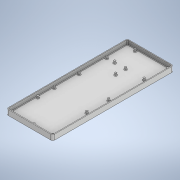
# Autodesk Inventor part: Base
Saved by Autodesk Inventor 2022 (Build 260153000, 153)
## iProperties
Created: 2021-09-21
Part Number: Base
Material: 一般
Document SubType Name: Modeling
Designer: shiok
Density: 1 g/cm^3
Appearance: 既定
Author: shiok
Autodesk Inventor part; units mm, degrees
ref_plane "YZ Plane" through (0, 0, 0) normal (1, 0, 0) x (0, 1, 0)
ref_plane "XZ Plane" through (0, 0, 0) normal (0, 1, 0) x (-1, 0, 0)
ref_plane "XY Plane" through (0, 0, 0) normal (0, 0, 1) x (1, 0, 0)
sketch "スケッチ1" plane through (0, 0, 0) normal (0, 1, 0) x (-1, 0, 0)
  line L0 (65.58, 183.1975) -> (-65.58, 183.1975)
  line L1 (-68.58, 180.1975) -> (-68.58, -180.1975)
  line L2 (-65.58, -183.1975) -> (65.58, -183.1975)
  line L3 (68.58, -180.1975) -> (68.58, 180.1975)
  arc A0 (68.58, 180.1975) -> (65.58, 183.1975) centre (65.58, 180.1975) ccw
  arc A1 (65.58, -183.1975) -> (68.58, -180.1975) centre (65.58, -180.1975) ccw
  arc A2 (-68.58, -180.1975) -> (-65.58, -183.1975) centre (-65.58, -180.1975) ccw
  arc A3 (-65.58, 183.1975) -> (-68.58, 180.1975) centre (-65.58, 180.1975) ccw
  line L4 (71.12, 180.1975) -> (71.12, -180.1975)
  arc A4 (65.58, -185.7375) -> (71.12, -180.1975) centre (65.58, -180.1975) ccw
  line L5 (65.58, -185.7375) -> (-65.58, -185.7375)
  arc A5 (-71.12, -180.1975) -> (-65.58, -185.7375) centre (-65.58, -180.1975) ccw
  line L6 (-71.12, -180.1975) -> (-71.12, 180.1975)
  arc A6 (-65.58, 185.7375) -> (-71.12, 180.1975) centre (-65.58, 180.1975) ccw
  line L7 (-65.58, 185.7375) -> (65.58, 185.7375)
  arc A7 (71.12, 180.1975) -> (65.58, 185.7375) centre (65.58, 180.1975) ccw
  line L8 (-65.58, 180.1975) -> (65.58, -180.1975) construction
  line L9 (-65.58, -180.1975) -> (65.58, 180.1975) construction
  circle A8 centre (62.23, 176.8475) radius 3
  circle A9 centre (63.5, 96.8375) radius 3
  circle A10 centre (63.5, 46.0375) radius 3
  circle A11 centre (62.23, -28.8925) radius 3
  circle A12 centre (62.23, -113.9825) radius 3
  circle A13 centre (38.1, -113.9825) radius 3
  circle A14 centre (38.1, -176.8475) radius 3
  circle A15 centre (-62.23, -176.8475) radius 3
  circle A16 centre (4.445, -113.9825) radius 3
  circle A17 centre (4.445, -83.5025) radius 3
  circle A18 centre (-52.705, -113.9825) radius 3
  circle A19 centre (-52.705, -4.7625) radius 3
  circle A20 centre (-52.705, 62.4375) radius 3
  circle A21 centre (-62.23, 176.8475) radius 3
  circle A22 centre (-5.08, 176.8475) radius 3
  point P0 (0, 0)
  point P1 (0, 0)
  point P2 (0, 0)
  point P3 (52.07, 166.6875)
  dimension "d2" = 3
  dimension "d3" = 2.54
  dimension "d5" = 366.395
  dimension "d6" = 137.16
  dimension "d7" = 16.51
  dimension "d8" = 16.51
  dimension "d9" = 10.16
  dimension "d10" = 10.16
  dimension "d11" = 1.27
  dimension "d12" = 1.27
  dimension "d13" = 80.01
  dimension "d14" = 50.8
  dimension "d15" = 74.93
  dimension "d16" = 85.09
  dimension "d17" = 6
  dimension "d18" = 6
  dimension "d19" = 6
  dimension "d20" = 6
  dimension "d21" = 6
  dimension "d22" = 24.13
  dimension "d23" = 62.865
  dimension "d24" = 100.33
  dimension "d25" = 62.865
  dimension "d26" = 9.525
  dimension "d27" = 6
  dimension "d28" = 6
  dimension "d29" = 57.15
  dimension "d30" = 67.2
  dimension "d31" = 6
  dimension "d32" = 6
  dimension "d33" = 109.22
  dimension "d34" = 6
  dimension "d35" = 6
  dimension "d36" = 6
  dimension "d37" = 6
  dimension "d38" = 6
  dimension "d39" = 6
  dimension "d40" = 30.48
  dimension "d41" = 33.655
  constraints: 23 centre point, 20 end point, 16 point on circle, 8 tangent, 7 vertical alignment, 5 horizontal alignment, 4 parallel, 3 equal radius, 3 midpoint, 2 perpendicular, 1 coincident, 1 horizontal, 7 other
  measures "d2" radius of A0
  measures "d3" distance between parallel lines of L3 L4
  measures "d5" distance between parallel lines of L2 L0
  measures "d6" distance between parallel lines of L1 L3
  measures "d7" distance from line of point (52.07, 166.688) L3
  measures "d8" distance from line of L0 point (52.07, 166.688)
  measures "d9" horizontal distance of A8.centre point (52.07, 166.688)
  measures "d10" horizontal distance of point (52.07, 166.688) A8.centre
  measures "d11" horizontal distance of A9.centre A8.centre
  measures "d12" horizontal distance of A11.centre A10.centre
  measures "d13" vertical distance of A9.centre A8.centre
  measures "d14" distance of A9.centre A10.centre
  measures "d15" vertical distance of A10.centre A11.centre
  measures "d16" distance of A12.centre A11.centre
  measures "d17" diameter of A8
  measures "d18" diameter of A9
  measures "d19" diameter of A10
  measures "d20" diameter of A11
  measures "d21" diameter of A12
  measures "d22" distance of A13.centre A12.centre
  measures "d23" distance of A14.centre A13.centre
  measures "d24" distance of A15.centre A14.centre
  measures "d25" vertical distance of A18.centre A15.centre
  measures "d26" horizontal distance of A18.centre A15.centre
  measures "d27" diameter of A21
  measures "d28" diameter of A22
  measures "d29" distance of A21.centre A22.centre
  measures "d30" distance of A19.centre A20.centre
  measures "d31" diameter of A20
  measures "d32" diameter of A19
  measures "d33" distance of A18.centre A19.centre
  measures "d34" diameter of A13
  measures "d35" diameter of A14
  measures "d36" diameter of A15
  measures "d37" diameter of A18
  measures "d38" diameter of A17
  measures "d39" diameter of A16
  measures "d40" distance of A17.centre A16.centre
  measures "d41" distance of A13.centre A16.centre
extrude "押し出し1" add sketch "スケッチ1" along normal blind 10 contours A8 | A9 | A10 | A11 | A12 | A13 | A14 | A15 | A16 | A17 | A18 | A19 | A20 | A21 | A22
sketch "スケッチ2" plane through (-63.5, 0, 96.8375) normal (0, -1, 0) x (1, 0, 0)
  line L0 (-2.08, 86.36) -> (129.08, 86.36)
  line L1 (132.08, 83.36) -> (132.08, -277.035)
  line L2 (129.08, -280.035) -> (-2.08, -280.035)
  line L3 (-5.08, -277.035) -> (-5.08, 83.36)
  arc A0 (-5.08, -277.035) -> (-2.08, -280.035) centre (-2.08, -277.035) ccw
  arc A1 (129.08, -280.035) -> (132.08, -277.035) centre (129.08, -277.035) ccw
  arc A2 (132.08, 83.36) -> (129.08, 86.36) centre (129.08, 83.36) ccw
  arc A3 (-2.08, 86.36) -> (-5.08, 83.36) centre (-2.08, 83.36) ccw
  line L4 (-2.08, -277.035) -> (129.08, 83.36) construction
  line L5 (-2.08, 83.36) -> (129.08, -277.035) construction
  line L6 (129.08, 88.9) -> (-2.08, 88.9)
  arc A4 (-2.08, 88.9) -> (-7.62, 83.36) centre (-2.08, 83.36) ccw
  line L7 (-7.62, 83.36) -> (-7.62, -277.035)
  arc A5 (-7.62, -277.035) -> (-2.08, -282.575) centre (-2.08, -277.035) ccw
  line L8 (-2.08, -282.575) -> (129.08, -282.575)
  arc A6 (129.08, -282.575) -> (134.62, -277.035) centre (129.08, -277.035) ccw
  line L9 (134.62, -277.035) -> (134.62, 83.36)
  arc A7 (134.62, 83.36) -> (129.08, 88.9) centre (129.08, 83.36) ccw
  point P0 (63.5, -96.8375)
  point P1 (63.5, -96.8375)
  point P2 (63.5, -96.8375)
  dimension "d44" = 3
  dimension "d45" = 366.395
  dimension "d46" = 137.16
  dimension "d47" = 2.54
  constraints: 20 end point, 16 point on circle, 8 centre point, 8 tangent, 4 parallel, 3 equal radius, 3 midpoint, 2 perpendicular, 1 coincident, 1 horizontal, 7 other
  measures "d44" radius of A0
  measures "d45" distance between parallel lines of L0 L2
  measures "d46" distance between parallel lines of L1 L3
  measures "d47" distance between parallel lines of L0 L6
extrude "押し出し2" add sketch "スケッチ2" against normal blind 15.8514
sketch "スケッチ3" plane through (5.08, 0, 176.8475) normal (0, -1, 0) x (1, 0, 0)
  line L0 (60.5, 6.35) -> (-70.66, 6.35)
  line L1 (-73.66, 3.35) -> (-73.66, -357.045)
  line L2 (-70.66, -360.045) -> (60.5, -360.045)
  line L3 (63.5, -357.045) -> (63.5, 3.35)
  arc A0 (-70.66, 6.35) -> (-73.66, 3.35) centre (-70.66, 3.35) ccw
  arc A1 (63.5, 3.35) -> (60.5, 6.35) centre (60.5, 3.35) ccw
  arc A2 (60.5, -360.045) -> (63.5, -357.045) centre (60.5, -357.045) ccw
  arc A3 (-73.66, -357.045) -> (-70.66, -360.045) centre (-70.66, -357.045) ccw
  line L4 (66.04, 3.35) -> (66.04, -357.045)
  arc A4 (60.5, -362.585) -> (66.04, -357.045) centre (60.5, -357.045) ccw
  line L5 (60.5, -362.585) -> (-70.66, -362.585)
  arc A5 (-76.2, -357.045) -> (-70.66, -362.585) centre (-70.66, -357.045) ccw
  line L6 (-76.2, -357.045) -> (-76.2, 3.35)
  arc A6 (-70.66, 8.89) -> (-76.2, 3.35) centre (-70.66, 3.35) ccw
  line L7 (-70.66, 8.89) -> (60.5, 8.89)
  arc A7 (66.04, 3.35) -> (60.5, 8.89) centre (60.5, 3.35) ccw
  line L8 (60.5, 3.35) -> (-70.66, -357.045) construction
  line L9 (60.5, -357.045) -> (-70.66, 3.35) construction
  point P0 (-5.08, -176.8475)
  point P1 (-5.08, -176.8475)
  point P2 (-5.08, -176.8475)
  dimension "d50" = 3
  dimension "d51" = 2.54
  dimension "d52" = 366.395
  dimension "d53" = 137.16
  constraints: 20 end point, 16 point on circle, 8 centre point, 8 tangent, 4 parallel, 3 equal radius, 3 midpoint, 2 perpendicular, 1 coincident, 1 horizontal, 7 other
  measures "d50" radius of A0
  measures "d51" distance between parallel lines of L3 L4
  measures "d52" distance between parallel lines of L2 L0
  measures "d53" distance between parallel lines of L3 L1
extrude "押し出し3" add sketch "スケッチ3" against normal blind 3.6 contours A1 L3 A2 L2 A3 L1 A0 L0 | L4 A4 L5 A5 L6 A6 L7 A7
fillet "フィレット1" radius 1.5 23 edges at (67.7013, 3.6, 182.3188) (0, 3.6, 183.1975) (-67.7013, 3.6, 182.3188) (-68.58, 3.6, 0) (-67.7013, 3.6, -182.3188) (0, 3.6, -183.1975) (67.7013, 3.6, -182.3188) (68.58, 3.6, 0) (65.23, 3.6, 176.8475) (8.08, 3.6, 176.8475) (55.705, 3.6, 62.4375) (55.705, 3.6, -4.7625) (-1.445, 3.6, -83.5025) (-1.445, 3.6, -113.9825) (55.705, 3.6, -113.9825) (65.23, 3.6, -176.8475) (-35.1, 3.6, -176.8475) (-35.1, 3.6, -113.9825) (-59.23, 3.6, -113.9825) (-59.23, 3.6, -28.8925) (-60.5, 3.6, 46.0375) (-60.5, 3.6, 96.8375) (-59.23, 3.6, 176.8475)
